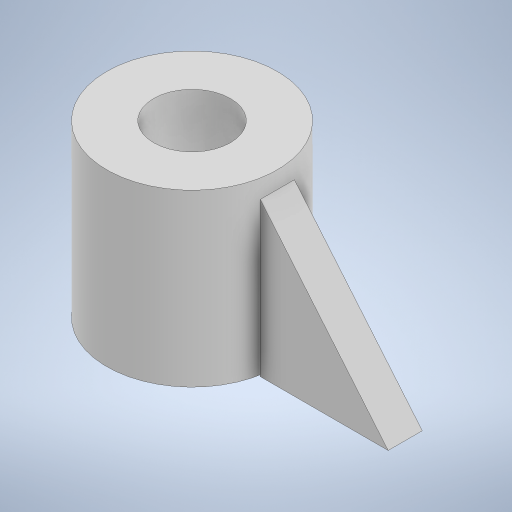
# Autodesk Inventor part: cilindro_obj2
Saved by Autodesk Inventor 2023.2 (Build 272271030, 271C)
## iProperties
Created: 2023-02-25
Part Number: cilindro_obj2
Material: Generic
Document SubType Name: Modeling
Designer: Cris Pat
Density: 1 g/cm^3
Appearance: Default
Author: Cris Pat
Autodesk Inventor part; units mm, degrees
ref_plane "YZ Plane" through (0, 0, 0) normal (1, 0, 0) x (0, 1, 0)
ref_plane "XY Plane" through (0, 0, 0) normal (0, 0, 1) x (1, 0, 0)
sketch "Sketch1" plane through (0, 0, 0) normal (0, 1, 0) x (-1, 0, 0)
  circle A0 centre (0, 0) radius 4.5
  circle A1 centre (0, 0) radius 10
  dimension "d0" = 9
  dimension "d1" = 20
  constraints: 2 centre point, 2 coincident
  measures "d0" diameter of A0
  measures "d1" diameter of A1
extrude "Extrusion1" add sketch "Sketch1" against normal blind 20 contours A0 | A1
extrude "Extrusion2" cut sketch "Sketch1" against normal blind 16 contours A0
sketch "Sketch2" plane through (0, 0, 0) normal (0, 0, 1) x (1, 0, 0)
  line L0 (-10, -20) -> (10, -20) construction
  line L1 (10, 0) -> (-10, 0) construction
  line L2 (10, -20) -> (25, -20)
  line L3 (25, -20) -> (10, -2)
  line L4 (10, -2) -> (10, -20)
  line L5 (10, 0) -> (10, -20) construction
  point P0 (0, 0)
  dimension "d6" = 15
  dimension "d7" = 18
  constraints: 6 end point, 1 collinear, 1 horizontal
  measures "d6" distance of L0.end L2.end
  measures "d7" distance of L0.end L3.end
extrude "Extrusion3" add sketch "Sketch2" along normal mid plane 4
ref_plane "Work Plane1" through (0, -16, 0) normal (0, 1, 0) x (-1, 0, 0)
sketch "Sketch3" plane through (0, -16, 0) normal (0, 1, 0) x (-1, 0, 0)
  circle A0 centre (0, 0) radius 2.75
  dimension "d11" = 5.5
  constraints: 1 centre point, 1 coincident
  measures "d11" diameter of A0
extrude "Extrusion4" cut sketch "Sketch3" against normal through all
body "Solid1"
